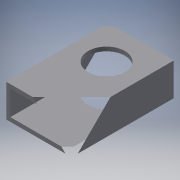
# Autodesk Inventor part: other end support
Saved by Autodesk Inventor 2016 (Build 200138000, 138)
## iProperties
Created: 2016-04-20
Part Number: other end support
Material: Generic
Document SubType Name: Modeling
Designer: gus
Density: 1 g/cm^3
Appearance: Default
Author: gus
Autodesk Inventor part; units mm, degrees
ref_plane "YZ Plane" through (0, 0, 0) normal (1, 0, 0) x (0, 1, 0)
ref_plane "XZ Plane" through (0, 0, 0) normal (0, 1, 0) x (-1, 0, 0)
ref_plane "XY Plane" through (0, 0, 0) normal (0, 0, 1) x (1, 0, 0)
sketch "Sketch1" plane through (0, 0, 0) normal (0, 0, 1) x (1, 0, 0)
  line L0 (0, 0) -> (-76.2, 0)
  line L1 (-76.2, 0) -> (-76.2, -25.4)
  line L2 (-76.2, -25.4) -> (0, -25.4)
  line L3 (0, -25.4) -> (0, 0)
  line L4 (-73.025, -22.225) -> (-73.025, -3.175)
  line L5 (-73.025, -3.175) -> (-3.175, -3.175)
  line L6 (-3.175, -3.175) -> (-3.175, -22.225)
  line L7 (-3.175, -22.225) -> (-73.025, -22.225)
  dimension "d0" = 76.2
  dimension "d1" = 25.4
  dimension "d2" = 3.175
  constraints: 16 end point, 4 parallel, 2 perpendicular, 1 horizontal, 3 other
  measures "d0" distance of L2.end L1.end
  measures "d1" distance of L1.end L0.end
  measures "d2" distance between parallel lines of L1 L4
extrude "Extrusion1" add sketch "Sketch1" along normal blind 79.375
sketch "Sketch2" plane through (-76.2, -25.4, 0) normal (0, -1, 0) x (1, 0, 0)
  circle A0 centre (40.7924, 38.1) radius 14.2875
  line L0 (0, 0) -> (76.2, 0) projected
  line L1 (76.2, 0) -> (76.2, 79.375) projected
  dimension "d5" = 28.575
  dimension "d6" = 38.1
  dimension "d7" = 35.4076
  constraints: 1 centre point
  measures "d5" diameter of A0
  measures "d6" distance from line of L0 A0.centre
  measures "d7" distance from line of A0.centre L1
extrude "Extrusion2" cut sketch "Sketch2" against normal blind 25.4
body "Solid1"
